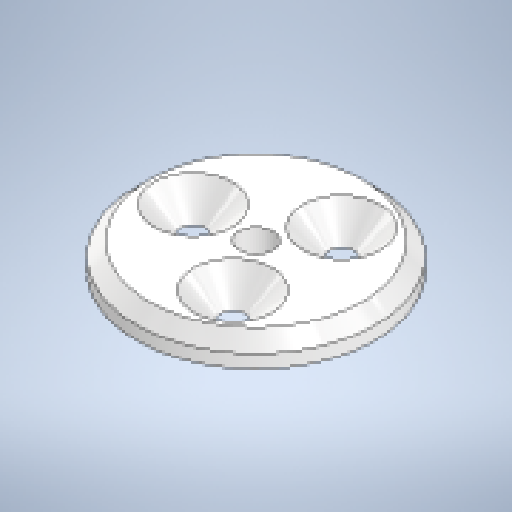
# Autodesk Inventor part: Hub Cap
Saved by Autodesk Inventor 2023.2 (Build 272271000, 271)
## iProperties
Created: 2023-06-14
Part Number: Hub Cap
Material: Nylon 6/6
Document SubType Name: Modeling
Designer: Nathan Cai
Density: 1.13 g/cm^3
Appearance: Smooth - White
Author: Nathan Cai
Autodesk Inventor part; units mm, degrees
ref_plane "YZ Plane" through (0, 0, 0) normal (1, 0, 0) x (0, 1, 0)
ref_plane "XZ Plane" through (0, 0, 0) normal (0, 1, 0) x (-1, 0, 0)
ref_plane "XY Plane" through (0, 0, 0) normal (0, 0, 1) x (1, 0, 0)
sketch "Sketch1" plane through (0, 0, 0) normal (0, 1, 0) x (-1, 0, 0)
  circle A0 centre (0, 0) radius 14.2875
  line L0 (0, 0) -> (14.2875, 0) construction
  dimension "d0" = 28.575
  constraints: 2 end point, 1 coincident, 1 horizontal, 1 horizontal alignment, 2 other
extrude "Extrusion1" add sketch "Sketch1" along normal blind 3.175
sketch "Sketch2" plane through (0, 3.175, 0) normal (0, 1, 0) x (1, 0, 0)
  circle A0 centre (0, 0) radius 2
  line L0 (0, 0) -> (-14.2875, 0) construction
  arc A1 (-12.8229, 3.4359) -> (-12.8229, -3.4359) centre (-9.525, 0) ccw projected
  circle A2 centre (0, 0) radius 7.5 construction
  circle A3 centre (-7.5, 0) radius 1.5
  circle A4 centre (3.75, -6.4952) radius 1.5
  circle A5 centre (3.75, 6.4952) radius 1.5
  dimension "d10" = 15
  dimension "d9" = 4
  dimension "d11" = 3
  dimension "d14" = 360
  constraints: 4 centre point, 2 coincident, 2 end point, 1 horizontal, 1 horizontal alignment, 1 point on circle, 1 point on line, 9 other
  measures "d9" diameter of A0
  measures "d11" diameter of A3
extrude "Extrusion2" cut sketch "Sketch2" against normal through all
chamfer "Chamfer1" distance 3.175 angle 45 3 edges at (-9, 3.175, 0) (2.25, 3.175, -6.4952) (2.25, 3.175, 6.4952)
chamfer "Chamfer2" distance 1.5875 angle 45 1 edges at (14.2875, 3.175, 0)
body "Solid1"
